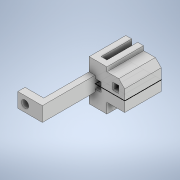
# Autodesk Inventor part: power and ground splitter holders
Saved by Autodesk Inventor 2022 (Build 260153000, 153)
## iProperties
Created: 2022-04-13
Part Number: power and ground splitter holders
Material: Generic
Document SubType Name: Modeling
Designer: a-dubs
Density: 1 g/cm^3
Appearance: Default
Author: a-dubs
Autodesk Inventor part; units mm, degrees
ref_plane "YZ Plane" through (0, 0, 0) normal (1, 0, 0) x (0, 1, 0)
ref_plane "XZ Plane" through (0, 0, 0) normal (0, 1, 0) x (-1, 0, 0)
ref_plane "XY Plane" through (0, 0, 0) normal (0, 0, 1) x (1, 0, 0)
sketch "Sketch1" plane through (0, 0, 0) normal (0, 1, 0) x (-1, 0, 0)
  line L0 (0, 0) -> (-2.6, 0)
  line L1 (-2.6, 0) -> (-2.6, -13.5)
  line L2 (-2.6, 0) -> (-3.6568, 0)
  line L3 (-2.6, -13.5) -> (0, -13.5)
  line L4 (0, -13.5) -> (0, 0)
  line L5 (0, 0) -> (0, 2.6)
  line L6 (0, 2.6) -> (-2.6, 2.6)
  line L7 (-2.6, 2.6) -> (-2.6, 0)
  line L8 (-2.6, 0) -> (-5.2, 0)
  line L9 (-5.2, 0) -> (-5.2, 2.6)
  line L10 (-5.2, 2.6) -> (-2.6, 2.6)
  line L11 (0, 0) -> (2.6, 0)
  line L12 (2.6, 0) -> (2.6, 2.6)
  line L13 (2.6, 2.6) -> (0, 2.6)
  line L14 (2.6, 0) -> (2.6, -13.5)
  line L15 (2.6, -13.5) -> (0, -13.5)
  line L16 (-2.6, -13.5) -> (-5.2, -13.5)
  line L17 (-5.2, -13.5) -> (-5.2, 0)
  line L18 (-10.4, 0) -> (-7.8, 0)
  line L19 (-7.8, 0) -> (-7.8, -13.5)
  line L20 (-7.8, 0) -> (-6.7432, 0)
  line L21 (-7.8, -13.5) -> (-10.4, -13.5)
  line L22 (-10.4, -13.5) -> (-10.4, 0)
  line L23 (-10.4, 0) -> (-10.4, 2.6)
  line L24 (-10.4, 2.6) -> (-7.8, 2.6)
  line L25 (-7.8, 2.6) -> (-7.8, 0)
  line L26 (-7.8, 0) -> (-5.2, 0)
  line L27 (-5.2, 2.6) -> (-7.8, 2.6)
  line L28 (-10.4, 0) -> (-13, 0)
  line L29 (-13, 0) -> (-13, 2.6)
  line L30 (-13, 2.6) -> (-10.4, 2.6)
  line L31 (-13, 0) -> (-13, -13.5)
  line L32 (-13, -13.5) -> (-10.4, -13.5)
  line L33 (-7.8, -13.5) -> (-5.2, -13.5)
  dimension "d0" = 2.6
  dimension "d1" = 13.5
  dimension "d2" = 2.6
  dimension "d3" = 2.6
  dimension "d6" = 2.6
  constraints: 68 end point, 10 perpendicular, 10 symmetric about line, 5 horizontal, 4 point on line, 1 vertical
  measures "d0" distance of L0.start L0.end
  measures "d1" distance of L0.end L1.end
  measures "d2" distance of L0.start L5.end
  measures "d3" distance of L0.end L8.end
  measures "d6" distance of L0.start L11.end
extrude "Extrusion1" add sketch "Sketch1" along normal mid plane 18 contours L11 L14 L15 L4 | L0 L7 L6 L5 | L5 L13 L12 L11 | L1 L16 L17 L8 L2 | L2 L8 L9 L10 L7
extrude "Extrusion2" add sketch "Sketch1" along normal mid plane 9 contours L33 L19 L20 L26 L17 | L26 L20 L25 L27 L9 | L25 L18 L23 L24 | L32 L31 L28 L22 | L23 L28 L29 L30
sketch "Sketch2" plane through (5.2, 9, -13.5) normal (0, 0, -1) x (-1, 0, 0)
  line L0 (5.2, -9) -> (0, -9)
  circle A0 centre (0, -9) radius 1.45
  dimension "d10" = 5.2
  dimension "d11" = 2.9
  constraints: 2 end point, 1 centre point, 1 coincident, 1 horizontal
  measures "d10" distance of L0.start L0.end
  measures "d11" diameter of A0
extrude "Extrusion3" cut sketch "Sketch2" against normal blind 6.4
sketch "Sketch3" plane through (2.6, 9, 0) normal (0, 0, -1) x (-1, 0, 0)
  line L0 (2.6, -9) -> (2.6, -11)
  line L1 (2.6, -18) -> (2.6, 0) projected
  line L2 (2.6, -11) -> (0, -11)
  line L3 (0, -18) -> (0, 0) projected
  line L4 (2.6, -9) -> (2.6, -7)
  line L5 (2.6, -7) -> (0, -7)
  line L6 (0, -7) -> (0, -11)
  point P0 (0, -7)
  dimension "d14" = 2
  dimension "d15" = 2
  constraints: 10 end point, 3 perpendicular, 3 point on line
  measures "d14" distance of L0.start L0.end
  measures "d15" distance of L0.start L4.end
sketch "Sketch4" plane through (10.4, 4.5, 0) normal (0, 0, -1) x (-1, 0, 0)
  line L0 (2.6, -9) -> (2.6, 0) projected
  line L1 (2.6, 0) -> (2.6, -3)
  line L2 (2.6, -3) -> (0, -3)
  line L3 (0, -9) -> (0, 0) projected
  line L4 (0, 0) -> (0, -3)
  line L5 (0, 0) -> (2.6, 0)
  line L6 (5.2, 0) -> (-2.6, 0) projected
  point P0 (10.4, -4.5)
  dimension "d16" = 3
  constraints: 8 end point, 2 collinear, 2 point on line, 1 perpendicular
  measures "d16" distance of L0.end L1.end
extrude "Extrusion4" add sketch "Sketch1" along normal blind 2.6 from surface at 4.5 contours L33 L19 L20 L26 L17 | L26 L20 L25 L27 L9 | L21 L22 L18 L19 | L25 L18 L23 L24 | L32 L31 L28 L22 | L23 L28 L29 L30
chamfer "Chamfer1" distance 2.6 angle 45 1 edges at (13, 7.1, -5.45)
extrude "Extrusion5" cut sketch "Sketch4" against normal through all
extrude "Extrusion6" cut sketch "Sketch3" against normal through all
sketch "Sketch5" plane through (-2.6, 9, 2.6) normal (0, 0, 1) x (1, 0, 0)
  line L0 (0, -18) -> (0, 0) projected
  line L1 (0, -9) -> (0, -5.8)
  line L2 (0, -5.8) -> (2.6, -5.8)
  line L3 (2.6, -5.8) -> (2.6, -12.2)
  line L4 (2.6, -12.2) -> (0, -12.2)
  line L5 (0, -12.2) -> (0, -5.8)
  point P0 (2.6, -9)
  dimension "d26" = 3.2
  dimension "d27" = 2.6
  dimension "d28" = 6.4
  constraints: 10 end point, 2 parallel, 1 horizontal, 1 midpoint, 1 perpendicular, 1 point on line
  measures "d26" distance of L1.start L1.end
  measures "d27" distance of L3.end L4.end
  measures "d28" distance of L2.end L3.end
extrude "Extrusion7" add sketch "Sketch5" along normal blind 20
sketch "Sketch6" plane through (-2.6, 9, 22.6) normal (0, 0, 1) x (1, 0, 0)
  line L0 (0, -5.8) -> (0, -12.2)
  line L1 (0, -5.8) -> (2.6, -5.8)
  line L2 (2.6, -5.8) -> (2.6, -12.2)
  line L3 (2.6, -5.8) -> (0, -5.8) projected
  line L4 (0, -5.8) -> (-1.8, -5.8)
  line L5 (-1.8, -5.8) -> (-1.8, -12.2)
  line L6 (-1.8, -12.2) -> (0, -12.2)
  line L7 (-1.8, -12.2) -> (-8.2, -12.2)
  line L8 (-8.2, -12.2) -> (-8.2, -5.8)
  line L9 (-8.2, -5.8) -> (-1.8, -5.8)
  line L10 (-1.8, -5.8) -> (-1.8, -12.2)
  circle A0 centre (-5, -9) radius 1.6
  point P0 (2.6, -9)
  point P1 (-1.8, -5.8)
  dimension "d32" = 6.4
  dimension "d38" = 1.8
  dimension "d39" = 6.4
  dimension "d40" = 3.2
  constraints: 20 end point, 3 perpendicular, 2 horizontal, 2 parallel, 1 centre point, 1 point on line
  measures "d32" distance of L0.start L0.end
  measures "d38" distance of L0.start L4.end
  measures "d39" distance of L8.end L9.end
  measures "d40" diameter of A0
extrude "Extrusion8" add sketch "Sketch6" along normal blind 3.2
extrude "Extrusion9" add sketch "Sketch5" along normal blind 3.2 from surface at 20
body "Solid1"
